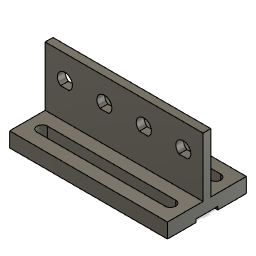
bnc_mount (Autodesk Fusion 360 design; units mm, degrees)
Autodesk Fusion 360 part; units mm, degrees
note: some values were not read from the file. Set by a fixed rule: which sketch regions a step uses.
sketch "Sketch1" plane through (0, 0, 0) normal (0, 1, 0) x (1, 0, 0)
  line L0 (-50.8, 25.4) -> (50.8, 25.4)
  line L1 (50.8, 25.4) -> (50.8, -25.4)
  line L2 (50.8, -25.4) -> (-50.8, -25.4)
  line L3 (-50.8, -25.4) -> (-50.8, 25.4)
  line L4 (-50.8, -25.4) -> (50.8, 25.4)
  line L5 (-50.8, 25.4) -> (50.8, -25.4)
  dimension "d1" = 50.8
  dimension "d2" = 101.6
  constraint horizontal L0
  constraint vertical L1
  constraint horizontal L2
  constraint vertical L3
  constraint coincident origin L4
  constraint coincident origin L5
  measures "d1" distance of L0.start L2.end
  measures "d2" distance of L1.end L2.end
extrude "Extrude1" add sketch "Sketch1" along normal blind 9.5
sketch "Sketch2" plane through (0, 9.5, 0) normal (0, 1, 0) x (-1, 0, 0)
  line L0 (50.8, 25.4) -> (-50.8, 25.4)
  line L1 (-50.8, 25.4) -> (-50.8, -25.4)
  line L2 (-50.8, -25.4) -> (50.8, -25.4)
  line L3 (50.8, -25.4) -> (50.8, 25.4)
  line L4 (50.8, -2.5) -> (-50.8, -2.5)
  line L5 (-50.8, -2.5) -> (-50.8, 2.5)
  line L6 (-50.8, 2.5) -> (50.8, 2.5)
  line L7 (50.8, 2.5) -> (50.8, -2.5)
  line L8 (50.8, 2.5) -> (-50.8, -2.5)
  dimension "d5" = 5
  constraint horizontal L4
  constraint vertical L5
  constraint horizontal L6
  constraint vertical L7
  constraint coincident L1 L5.end
  constraint coincident L3 L4.start
  constraint coincident origin L8
  measures "d5" distance of L4.end L5.end
extrude "Extrude2" add sketch "Sketch2" along normal blind 38.1 contours L1 L5 L6 L8 | L3 L4 L7 L8
sketch "Sketch3" plane through (0, 9.5, 0) normal (0, 1, 0) x (-1, 0, 0)
  line L0 (-50.8, 2.5) -> (50.8, 2.5)
  line L1 (50.8, 2.5) -> (50.8, 25.4)
  line L2 (50.8, 25.4) -> (-50.8, 25.4)
  line L3 (-50.8, 25.4) -> (-50.8, 2.5)
  line L4 (41.3, 10.575) -> (-41.3, 10.575)
  line L5 (-41.3, 10.575) -> (-41.3, 17.325)
  line L6 (-41.3, 17.325) -> (41.3, 17.325)
  line L7 (41.3, 17.325) -> (41.3, 10.575)
  line L8 (0, 2.5) -> (0, 10.575)
  line L9 (0, 17.325) -> (0, 25.4)
  line L10 (41.3, 13.95) -> (50.8, 13.95)
  line L11 (-41.3, 13.95) -> (-50.8, 13.95)
  line L12 (41.341, -18.4703) -> (-41.259, -18.4703)
  line L13 (-41.259, -18.4703) -> (-41.259, -11.7203)
  line L14 (-41.259, -11.7203) -> (41.341, -11.7203)
  line L15 (41.341, -11.7203) -> (41.341, -18.4703)
  line L16 (0.041, -26.5453) -> (0.041, -18.4703)
  dimension "d8" = 82.6
  dimension "d9" = 6.75
  constraint horizontal L4
  constraint vertical L5
  constraint horizontal L6
  constraint vertical L7
  constraint midpoint L0 L8.start
  constraint coincident L4 L8.end
  constraint perpendicular L4 L8
  constraint coincident L6 L9.start
  constraint midpoint L2 L9.end
  constraint perpendicular L2 L9
  constraint equal L8 L9
  constraint midpoint L7 L10.start
  constraint midpoint L1 L10.end
  constraint midpoint L5 L11.start
  constraint midpoint L3 L11.end
  constraint equal L10 L11
  constraint horizontal L12
  constraint vertical L13
  constraint horizontal L14
  constraint vertical L15
  constraint equal L4 L14
  constraint equal L7 L15
  constraint midpoint L12 L16.end
  constraint perpendicular L12 L16
  constraint equal L8 L16
  measures "d8" distance of L5.end L6.end
  measures "d9" distance of L4.start L6.end
extrude "Extrude3" cut sketch "Sketch3" against normal blind 20 contours L4 L5 L6 L7 | L12 L13 L14 L15
hole "Hole1" at (-41.3, 9.5, 13.95) direction (0, -1, 0) diameter 6.75 depth 30 tip angle 118
hole "Hole2" at (-41.341, 9.5, -15.0953) direction (0, -1, 0) diameter 6.75 depth 30 tip angle 118
hole "Hole3" at (41.259, 9.5, -15.0953) direction (0, -1, 0) diameter 6.75 depth 30 tip angle 118
hole "Hole4" at (41.3, 9.5, 13.95) direction (0, -1, 0) diameter 6.75 depth 30 tip angle 118
sketch "Sketch4" plane through (0, 0, 0) normal (0, -1, 0) x (1, 0, 0)
  arc A0 (41.259, -18.4703) -> (41.259, -11.7203) centre (41.259, -15.0953) ccw
  line L0 (41.259, -18.4703) -> (-41.341, -18.4703)
  arc A1 (-41.341, -11.7203) -> (-41.341, -18.4703) centre (-41.341, -15.0953) ccw
  line L1 (-41.341, -11.7203) -> (41.259, -11.7203)
  arc A2 (41.3, 10.575) -> (41.3, 17.325) centre (41.3, 13.95) ccw
  line L2 (41.3, 10.575) -> (-41.3, 10.575)
  arc A3 (-41.3, 17.325) -> (-41.3, 10.575) centre (-41.3, 13.95) ccw
  line L3 (-41.3, 17.325) -> (41.3, 17.325)
  line L4 (50.8, 25.4) -> (-50.8, 25.4)
  line L5 (-50.8, 25.4) -> (-50.8, -25.4)
  line L6 (-50.8, -25.4) -> (50.8, -25.4)
  line L7 (50.8, -25.4) -> (50.8, 25.4)
  line L8 (-50.8, 7) -> (50.8, 7)
  line L9 (50.8, 7) -> (50.8, -7)
  line L10 (50.8, -7) -> (-50.8, -7)
  line L11 (-50.8, -7) -> (-50.8, 7)
  line L12 (-50.8, 0) -> (50.8, 0)
  line L13 (0, 7) -> (0, -7)
  dimension "d25" = 101.6
  dimension "d26" = 14
  constraint horizontal L8
  constraint vertical L9
  constraint horizontal L10
  constraint vertical L11
  constraint midpoint L11 L12.start
  constraint midpoint L9 L12.end
  constraint midpoint L8 L13.start
  constraint midpoint L10 L13.end
  constraint midpoint origin L12
  measures "d25" distance of L8.start L8.end
  measures "d26" distance of L8.end L9.end
extrude "Extrude4" cut sketch "Sketch4" against normal blind 2 contours L7 L8 L9 L12 L13 | L5 L8 L11 L12 L13 | L7 L9 L10 L12 L13 | L5 L10 L11 L12 L13
sketch "Sketch5" plane through (0, 0, -2.5) normal (0, 0, -1) x (-1, 0, 0)
  line L0 (-50.8, 9.5) -> (50.8, 9.5)
  line L1 (50.8, 9.5) -> (50.8, 47.6)
  line L2 (50.8, 47.6) -> (-50.8, 47.6)
  line L3 (-50.8, 47.6) -> (-50.8, 9.5)
  circle A0 centre (-38.1, 32.142) radius 4.85
  circle A1 centre (-12.7, 32.142) radius 4.8997
  circle A2 centre (12.7, 32.142) radius 4.85
  circle A3 centre (38.1, 32.142) radius 4.85
  line L4 (-38.1, 32.142) -> (-12.7, 32.142)
  line L5 (-12.7, 32.142) -> (12.7, 32.142)
  line L6 (12.7, 32.142) -> (38.1, 32.142)
  line L7 (-42.95, 37.0417) -> (42.95, 37.0417)
  line L8 (42.95, 37.0417) -> (42.95, 28.1917)
  line L9 (42.95, 28.1917) -> (-42.95, 28.1917)
  line L10 (-42.95, 28.1917) -> (-42.95, 37.0417)
  line L11 (42.95, 32.6167) -> (50.8, 32.6167)
  line L12 (-42.95, 32.6167) -> (-50.8, 32.6167)
  dimension "d29" = 9.7
  dimension "d31" = 8.85
  dimension "d32" = 25.4
  constraint equal A0 A3
  constraint coincident A0.centre L4.start
  constraint coincident A1.centre L4.end
  constraint coincident A2.centre L5.end
  constraint coincident A3.centre L6.end
  constraint parallel L2 L6
  constraint equal L4 L5
  constraint equal L5 L6
  constraint parallel L4 L5
  constraint parallel L5 L6
  constraint horizontal L7
  constraint vertical L8
  constraint horizontal L9
  constraint vertical L10
  constraint tangent A1 L7
  constraint tangent A0 L10
  constraint tangent A3 L8
  constraint midpoint L8 L11.start
  constraint coincident L1 L11.end
  constraint perpendicular L1 L11
  constraint midpoint L10 L12.start
  constraint coincident L3 L12.end
  constraint perpendicular L3 L12
  constraint equal L11 L12
  measures "d29" diameter of A0
  measures "d31" distance of L7.start L9.end
  measures "d32" distance of A0.centre A1.centre
extrude "Extrude5" cut sketch "Sketch5" against normal blind 20 contours A0 L9 | A3 L9 | A1 L4 L5 | A1 L4 L5 L9 | A2 L5 L6 | A2 L5 L6 L9 picked at (-39.4169, 32.3517) picked at (37.6141, 31.8651)
equation "d8 = 101.6 mm - 19 mm"
